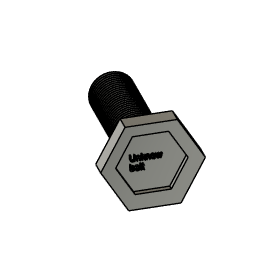
Day 4 bolt (Autodesk Fusion 360 design; units mm, degrees)
Autodesk Fusion 360 part; units mm, degrees
sketch "Sketch1" plane through (0, 0, 0) normal (0, 0, 1) x (1, 0, 0)
  line L0 (-76.8295, 22.5045) -> (-57.9042, -55.2841)
  line L1 (-57.9042, -55.2841) -> (18.9253, -77.7885)
  line L2 (18.9253, -77.7885) -> (76.8295, -22.5045)
  line L3 (76.8295, -22.5045) -> (57.9042, 55.2841)
  line L4 (57.9042, 55.2841) -> (-18.9253, 77.7885)
  line L5 (-18.9253, 77.7885) -> (-76.8295, 22.5045)
extrude "Extrude1" add sketch "Sketch1" along normal blind 30
sketch "Sketch2" plane through (0, 0, 30) normal (0, 0, 1) x (-1, 0, 0)
  line L0 (18.9253, -77.7885) -> (76.8295, -22.5045)
  line L1 (76.8295, -22.5045) -> (57.9042, 55.2841)
  line L2 (57.9042, 55.2841) -> (-18.9253, 77.7885)
  line L3 (-18.9253, 77.7885) -> (-76.8295, 22.5045)
  line L4 (-76.8295, 22.5045) -> (-57.9042, -55.2841)
  line L5 (-57.9042, -55.2841) -> (18.9253, -77.7885)
  circle A0 centre (0, 0) radius 36.0555
  constraint coincident A0.centre origin
extrude "Extrude2" add sketch "Sketch2" along normal blind 70 contours A0
extrude "Extrude3" add 1 faces at (5.9453, -7.96, 100) along direction (0, 0, 1) blind 150
thread "Thread1" "ISO Metric profile 72.0 M72x6 6g" major diameter 71.62 minor diameter 64.736 pitch 6 angle 60 modelled right hand crest width 0.8424 on face at (-36.0107, 1.7972, 176.6667) crest through (-35.81, 0, 28.5)
move_body "Move1" bodies 1 to x (0.523136, 0.499464, 0.690554) y (0.499464, 0.476864, -0.723281) z (-0.690554, 0.723281, 0) at (46.166, -108.9949, 14.4444)
move_body "Move2" bodies 1 to x (0.955306, 0.275984, 0.105941) y (-0.264825, 0.958209, -0.108182) z (-0.13137, 0.075292, 0.98847) at (-27.5551, -37.6704, 51.579)
sketch "Sketch3" plane through (97.0371, -57.2798, 17.2594) normal (0.851233, -0.502473, 0.151404) x (0.508333, 0.861161, 0)
  line L0 (-128.2453, -3.3686) -> (-48.1878, -3.2132)
  line L1 (-48.1878, -3.2132) -> (-8.2937, 66.1964)
  line L2 (-8.2937, 66.1964) -> (-48.457, 135.4505)
  line L3 (-48.457, 135.4505) -> (-128.5145, 135.295)
  line L4 (-128.5145, 135.295) -> (-168.4087, 65.8855)
  line L5 (-168.4087, 65.8855) -> (-128.2453, -3.3686)
  line L6 (-34.5806, 70.2714) -> (-62.5253, 118.1303)
  line L7 (-62.5253, 118.1303) -> (-117.9447, 117.8589)
  line L8 (-117.9447, 117.8589) -> (-145.4194, 69.7286)
  line L9 (-145.4194, 69.7286) -> (-117.4747, 21.8697)
  line L10 (-117.4747, 21.8697) -> (-62.0553, 22.1411)
  line L11 (-62.0553, 22.1411) -> (-34.5806, 70.2714)
  point P0 (-90, 70)
extrude "Extrude4" cut sketch "Sketch3" against normal blind 10 contours L6 L7 L8 L9 L10 L11
sketch "Sketch4" plane through (88.5247, -52.2551, 15.7454) normal (0.851233, -0.502473, 0.151404) x (0.508333, 0.861161, 0)
  line L0 (-62.0553, 22.1411) -> (-34.5806, 70.2714)
  line L1 (-34.5806, 70.2714) -> (-62.5253, 118.1303)
  line L2 (-62.5253, 118.1303) -> (-117.9447, 117.8589)
  line L3 (-117.9447, 117.8589) -> (-145.4194, 69.7286)
  line L4 (-145.4194, 69.7286) -> (-117.4747, 21.8697)
  line L5 (-117.4747, 21.8697) -> (-62.0553, 22.1411)
  line L6 (-121.5946, 62.0318) -> (-54.9336, 62.0318) construction
  line L7 (-54.9336, 62.0318) -> (-54.9336, 83.6349) construction
  line L8 (-54.9336, 83.6349) -> (-121.5946, 83.6349) construction
  line L9 (-121.5946, 83.6349) -> (-121.5946, 62.0318) construction
  dimension "d11" = 10
  text T0 "Unknow bolt" font "Arial" height 10 align left top in box 66.661 x 21.6031 at (-121.5946, 62.0318) x (1, 0) y (0, 1) spacing 1 kerned
extrude "Extrude5" add sketch "Sketch4" along normal blind 5 text T0
